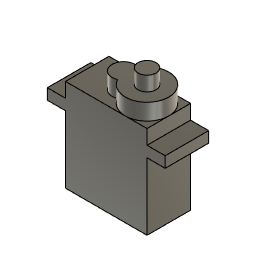
Engine Nozzle Version 3 v139 (Autodesk Fusion 360 archive; units mm, degrees)
design "MG90S SERVOMOTOR"
Autodesk Fusion 360 part; units mm, degrees
sketch "Sketch1" plane through (0, 0, 0) normal (0, 1, 0) x (1, 0, 0)
  line L0 (0, 0) -> (5, 0)
  line L1 (5, 0) -> (27.5, 0)
  line L2 (27.5, 0) -> (27.5, -18.5)
  line L3 (5, -18.5) -> (5, 0)
  line L4 (5, -21.5) -> (0, -21.5)
  line L5 (0, -21.5) -> (0, -18.5)
  line L6 (0, -18.5) -> (5, -18.5)
  line L7 (27.5, -21.5) -> (32.5, -21.5)
  line L8 (32.5, -21.5) -> (32.5, -18.5)
  line L9 (32.5, -18.5) -> (27.5, -18.5)
  line L10 (27.5, -21.5) -> (27.5, -25.5)
  line L11 (27.5, -25.5) -> (5, -25.5)
  line L12 (5, -25.5) -> (5, -21.5)
  dimension "d1" = 5
  dimension "d2" = 22.5
  dimension "d3" = 18.5
  dimension "d4" = 3
  dimension "d5" = 5
  dimension "d6" = 3
  dimension "d7" = 5
  dimension "d8" = 22.5
  dimension "d9" = 4
  constraint coincident L0.start origin
  constraint horizontal L0
  constraint horizontal L1
  constraint vertical L2
  constraint vertical L3
  constraint horizontal L4
  constraint vertical L5
  constraint horizontal L6
  constraint horizontal L7
  constraint vertical L8
  constraint horizontal L9
  constraint vertical L10
  constraint horizontal L11
  constraint vertical L12
  measures "d1" distance of L0.start L0.end
  measures "d2" distance of L0.end L1.end
  measures "d3" distance of L0.end L3.start
  measures "d4" distance of L3.start L4.start
  measures "d5" distance of L4.start L4.end
  measures "d6" distance of L4.start L3.start
  measures "d7" distance of L7.start L7.end
  measures "d8" distance of L4.start L7.start
  measures "d9" distance of L4.start L11.end
extrude "Extrude1" add sketch "Sketch1" along normal blind 12
sketch "Sketch2" plane through (0, 0, 25.5) normal (0, 0, 1) x (-1, 0, 0)
  line L0 (-5, 0) -> (-27.5, 0)
  line L1 (-27.5, 0) -> (-27.5, -12)
  line L2 (-27.5, -12) -> (-5, -12)
  line L3 (-5, -12) -> (-5, 0)
  circle A0 centre (-21.5, -6) radius 6
  circle A1 centre (-15, -6) radius 3.15
  dimension "d14" = 6.3
  constraint tangent L2 A0
  constraint tangent L1 A0
  constraint tangent L0 A0
  measures "d14" diameter of A1
extrude "Extrude2" add sketch "Sketch2" along normal blind 4.5 contours A0 A1 | A0 A1 picked at (-24.363, -5.7154) picked at (-16.388, -6.4033)
extrude "Extrude3" add sketch "Sketch2" along normal blind 4.5 contours A0 A1 picked at (-14.3919, -6.6826)
sketch "Sketch3" plane through (0, 0, 30) normal (0, 0, 1) x (-1, 0, 0)
  arc A0 (-16.244, -3.1061) -> (-16.244, -8.8939) centre (-21.5, -6) ccw
  arc A1 (-16.244, -8.8939) -> (-16.244, -3.1061) centre (-15, -6) ccw
  circle A2 centre (-21.5, -6) radius 2.5
  dimension "d17" = 5
  constraint concentric A0 A2
  measures "d17" diameter of A2
extrude "Extrude4" add sketch "Sketch3" along normal blind 4 contours A2
